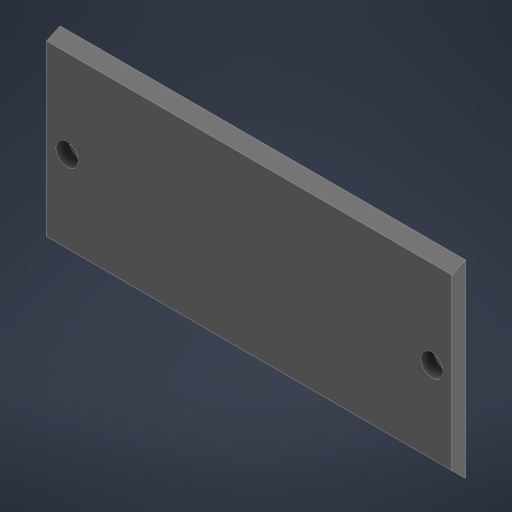
# Autodesk Inventor part: pług_część2
Saved by Autodesk Inventor 2023.4 (Build 274418000, 418)
## iProperties
Created: 2025-10-31
Part Number: pług_część2
Material: Stal
Document SubType Name: Modeling
Designer: Jakub Borsukiewicz
Density: 7.85 g/cm^3
Appearance: Szara
Author: Jakub Borsukiewicz
Autodesk Inventor part; units mm, degrees
ref_plane "YZ Plane" through (0, 0, 0) normal (1, 0, 0) x (0, 1, 0)
ref_plane "XZ Plane" through (0, 0, 0) normal (0, 1, 0) x (-1, 0, 0)
ref_plane "XY Plane" through (0, 0, 0) normal (0, 0, 1) x (1, 0, 0)
sketch "Szkic1" plane through (0, 0, 0) normal (0, 0, 1) x (1, 0, 0)
  line L0 (-63, 0) -> (63, 0) projected
  line L1 (0, -29.4) -> (0, 29.4) projected
  line L2 (-45, -21) -> (45, -21)
  line L3 (45, -21) -> (45, 21)
  line L4 (45, 21) -> (-45, 21)
  line L5 (-45, 21) -> (-45, -21)
  line L6 (-45, -21) -> (45, 21) construction
  line L7 (45, -21) -> (-45, 21) construction
  point P0 (0, 0)
  dimension "d0" = 90
  dimension "d1" = 42
  constraints: 12 end point, 2 midpoint, 2 parallel, 1 horizontal, 1 perpendicular
  measures "d0" distance of L3.end L4.end
  measures "d1" distance of L2.end L3.end
extrude "Wyciągnięcie proste1" add sketch "Szkic1" along normal blind 3
sketch "Szkic2" plane through (45, -21, 0) normal (1, 0, 0) x (0, 0, -1)
  line L0 (0, 0) -> (0, 42) projected
  line L1 (0, 42) -> (-3, 42) projected
  line L2 (-3, 0) -> (-3, 42) projected
  line L3 (0, 0) -> (-3, 0) projected
  line L4 (0, 0) -> (-3, 0) projected
  line L5 (0, 0) -> (-3, 3)
  line L6 (-3, 0) -> (-3, 42) projected
  line L7 (0, 42) -> (-3, 42) projected
  line L8 (0, 42) -> (-3, 40.6011)
  point P0 (0, 21)
  dimension "d4" = 45
  dimension "d5" = 65
  constraints: 4 end point, 2 point on line
  measures "d4" angle of L0 L5
  measures "d5" angle of L0 L8
extrude "Wyciągnięcie proste2" cut sketch "Szkic2" against normal blind 90 contours L3 L2 L5 | L8 L2 L1
sketch "Szkic3" plane through (0, 0, 0) normal (0, 0, -1) x (-1, 0, 0)
  line L0 (45, 21) -> (45, -21) projected
  line L1 (-45, 21) -> (45, 21) projected
  point P0 (0, 0)
  point P1 (40.5, 0)
  dimension "d8" = 4.5
  dimension "d9" = 21
  measures "d8" distance from line of L0 point (40.5, 0)
  measures "d9" distance from line of L1 point (40.5, 0)
hole "Otwór1" at (-40.5, 0, 0) direction (0, 0, 1) diameter 5 depth 4
mirror "Odbij1" about plane through (0, 0, 0) normal (1, 0, 0) of "Otwór1"
